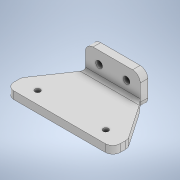
# Autodesk Inventor part: CameraHolder
Saved by Autodesk Inventor 2020 (Build 240168000, 168)
## iProperties
Created: 2023-05-25
Part Number: CameraHolder
Material: Generic
Document SubType Name: Modeling
Designer: DSOB
Density: 1 g/cm^3
Appearance: Default
Author: DSOB
Autodesk Inventor part; units mm, degrees
ref_plane "YZ Plane" through (0, 0, 0) normal (1, 0, 0) x (0, 1, 0)
ref_plane "XZ Plane" through (0, 0, 0) normal (0, 1, 0) x (-1, 0, 0)
ref_plane "XY Plane" through (0, 0, 0) normal (0, 0, 1) x (1, 0, 0)
sketch "Sketch1" plane through (0, 0, 0) normal (0, 0, 1) x (1, 0, 0)
  line L0 (0, 0) -> (36, 0)
  line L1 (36, 0) -> (36, 16)
  line L2 (36, 16) -> (0, 16)
  line L3 (0, 16) -> (0, 0)
  dimension "d0" = 36
  dimension "d1" = 16
  constraints: 8 end point, 2 parallel, 1 horizontal, 1 perpendicular
  measures "d0" distance of L1.end L2.end
  measures "d1" distance of L0.end L1.end
extrude "Extrusion1" add sketch "Sketch1" along normal blind 5
sketch "Sketch2" plane through (0, 0, 5) normal (0, 0, 1) x (1, 0, 0)
  circle A0 centre (9, 8) radius 2.25
  circle A1 centre (27, 8) radius 2.25
  line L0 (0, 0) -> (36, 0) projected
  line L1 (0, 16) -> (0, 0) projected
  dimension "d4" = 4.5
  dimension "d5" = 4.5
  dimension "d6" = 8
  dimension "d7" = 0
  dimension "d8" = 18
  dimension "d9" = 9
  constraints: 2 centre point
  measures "d4" diameter of A0
  measures "d5" diameter of A1
  measures "d6" distance from line of L0 A0.centre
  measures "d7" vertical distance of A0.centre A1.centre
  measures "d8" distance of A1.centre A0.centre
  measures "d9" distance from line of L1 A0.centre
extrude "Extrusion2" cut sketch "Sketch2" against normal blind 5
sketch "Sketch3" plane through (0, 0, 0) normal (0, -1, 0) x (1, 0, 0)
  line L0 (0, 0) -> (36, 0) projected
  line L1 (0, 0) -> (0, 5) projected
  line L2 (0, 0) -> (0, 5)
  line L3 (0, 5) -> (-17, 30)
  line L4 (-17, 30) -> (-17, 40)
  line L5 (-17, 40) -> (53, 40)
  line L6 (53, 40) -> (53, 30)
  line L7 (36, 5) -> (0, 5) projected
  line L8 (53, 30) -> (36, 5)
  line L9 (36, 0) -> (36, 5) projected
  line L10 (36, 5) -> (36, 0)
  line L11 (36, 0) -> (0, 0)
  circle A0 centre (-4.4, 32) radius 1.75
  circle A1 centre (40.4, 32) radius 1.75
  dimension "d12" = 40
  dimension "d13" = 70
  dimension "d14" = 10
  dimension "d15" = 10
  dimension "d16" = 17
  dimension "d17" = 3.5
  dimension "d18" = 3.5
  dimension "d19" = 44.8
  dimension "d20" = 0
  dimension "d21" = 4.4
  dimension "d22" = 32
  constraints: 16 end point, 3 perpendicular, 2 centre point, 2 parallel, 1 collinear
  measures "d12" distance between parallel lines of L0 L5
  measures "d13" distance of L4.end L5.end
  measures "d14" distance of L3.end L4.end
  measures "d15" distance of L5.end L6.end
  measures "d16" distance between parallel lines of L1 L4
  measures "d17" diameter of A0
  measures "d18" diameter of A1
  measures "d19" distance of A1.centre A0.centre
  measures "d20" vertical distance of A1.centre A0.centre
  measures "d21" distance from line of L1 A0.centre
  measures "d22" distance from line of L0 A0.centre
extrude "Extrusion3" add sketch "Sketch3" along normal blind 5
fillet "Fillet1" radius 2 1 edges at (18, 0, 5)
fillet "Fillet2" radius 5 2 edges at (36, 16, 2.5) (0, 16, 2.5)
fillet "Fillet3" radius 5 2 edges at (36, -5, 2.5) (0, -5, 2.5)
fillet "Fillet4" radius 5 4 edges at (53, -2.5, 40) (-17, -2.5, 40) (53, -2.5, 30) (-17, -2.5, 30)
body "Solid1"
